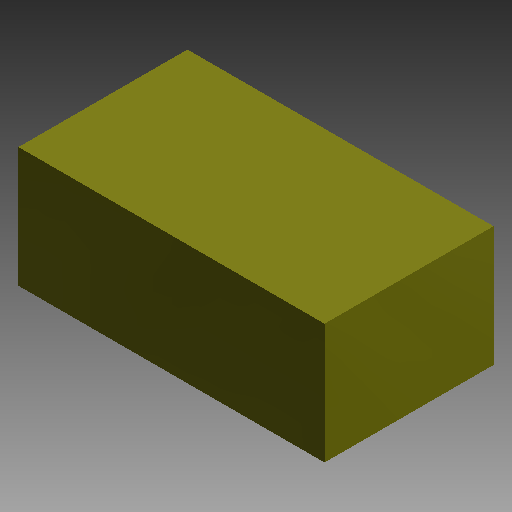
# Autodesk Inventor part: 0395311004
Saved by Autodesk Inventor 2018.2 (Build 222227000, 227)
## iProperties
Part Number: 0395311004
Material: Generic
Document SubType Name: Modeling
Designer: autocad
Appearance: MSTBV4, 0395311004
Author: autocad
Autodesk Inventor part; units mm, degrees
ref_plane "YZ Plane" through (0, 0, 0) normal (1, 0, 0) x (0, 1, 0)
ref_plane "XZ Plane" through (0, 0, 0) normal (0, 1, 0) x (-1, 0, 0)
ref_plane "XY Plane" through (0, 0, 0) normal (0, 0, 1) x (1, 0, 0)
sketch "MSTBV4, 0395311004_118" plane through (0, 0, 0) normal (0, 0, 1) x (1, 0, 0)
  line L0 (-10.8712, -3.8862) -> (-10.8712, 4.6482)
  line L1 (-10.8712, 4.6482) -> (10.8712, 4.6482)
  line L2 (10.8712, 4.6482) -> (10.8712, -3.8862)
  line L3 (10.8712, -3.8862) -> (-10.8712, -3.8862)
  constraints: 8 end point
extrude "Extrusion1" add sketch "MSTBV4, 0395311004_118" along normal blind 12
body "Solid1"
